DHECbottomlockcapv2 (Autodesk Fusion 360 design; units mm, degrees)
Autodesk Fusion 360 part; units mm, degrees
note: some values were not read from the file. Chosen so that the rebuilt part matches the saved one: a direction. Set by a fixed rule: which sketch regions a step uses.
sketch "Sketch1" plane through (0, 0, 0) normal (0, 0, 1) x (1, 0, 0)
  circle A0 centre (0, 0) radius 37.5
  dimension "d1" = 75
  constraint coincident A0.centre origin
  measures "d1" diameter of A0
extrude "Extrude1" add sketch "Sketch1" along normal blind 5
sketch "Sketch2" plane through (0, 0, 0) normal (1, 0, 0) x (0, 1, 0)
  line L0 (-6.5, 5) -> (-6.5, 15)
  line L1 (6.5, 5) -> (6.5, 15)
  circle A0 centre (0, 15) radius 6.5
  line L2 (0, 1.75) -> (0, 22.5)
  line L3 (37.5, 5) -> (-37.5, 5)
  line L4 (-10, 5) -> (-10, 15)
  circle A1 centre (0, 15) radius 10
  line L5 (10, 5) -> (10, 15)
  line L6 (-10, 15) -> (-6.5, 15)
  line L7 (10, 15) -> (6.5, 15)
  circle A2 centre (0, 15) radius 3.5
  dimension "d4" = 13
  dimension "d5" = 10
  dimension "d6" = 20
  dimension "d14" = 7
  constraint vertical L0
  constraint vertical L1
  constraint coincident L1.end A0
  constraint tangent L1 A0
  constraint tangent L0 A0
  constraint coincident A0.centre L2
  constraint coincident L3 L4.start
  constraint perpendicular L3 L4
  constraint concentric A0 A1
  constraint coincident L4.end A1
  constraint coincident L3 L5.start
  constraint coincident A1 L5.end
  constraint tangent A1 L5
  constraint vertical L5
  constraint horizontal L4.end A0.centre
  constraint perpendicular L0 L6
  constraint concentric A0 A2
  measures "d4" diameter of A0
  measures "d5" distance of A0.centre L3
  measures "d6" diameter of A1
  measures "d14" diameter of A2
extrude "Extrude2" add sketch "Sketch2" along normal mid plane 35 contours L0 L3 L4 A1 | L0 L3 A1 | L0 A1 L6 | L0 A0 L2 A1 | L1 L3 A1 | L1 A0 L2 A1 | L1 L3 A1 L5 | L1 A1 L7
extrude "Extrude3" add sketch "Sketch2" along normal blind 5 from surface at 17.5 contours L0 L3 L4 A1 | L0 L3 A1 | L0 A1 L6 | L0 A0 L2 A1 | L1 L3 A1 | L1 A0 L2 A1 | A0 A1 L6 L7 | A0 L2 A2 | A0 L2 A2 | L1 L3 A1 L5 | L1 A1 L7
mirror "Mirror1" about plane through (0, 0, 0) normal (1, 0, 0) of "Extrude3"
sketch "Sketch3" plane through (0, 0, 0) normal (0, 1, 0) x (1, 0, 0)
sketch "Sketch4" plane through (0, 0, 5) normal (0, 0, 1) x (-1, 0, 0)
  circle A0 centre (0, 0) radius 37.5
  line L0 (-22.5, 10) -> (22.5, 10)
  line L1 (22.5, 10) -> (22.5, -10)
  line L2 (22.5, -10) -> (-22.5, -10)
  line L3 (-22.5, -10) -> (-22.5, 10)
  circle A1 centre (0, 32.5) radius 5
  line L4 (5, 32.5) -> (5, 37.1652)
  line L5 (-5, 32.5) -> (-5, 37.1652)
  dimension "d15" = 10
  constraint tangent A0 A1
  constraint vertical A1.centre A0.centre
  constraint coincident A1 L4.start
  constraint coincident A0 L4.end
  constraint coincident A1 L5.start
  constraint coincident A0 L5.end
  constraint tangent A1 L5
  constraint tangent A1 L4
  constraint parallel L4 L5
  constraint parallel L3 L4
  measures "d15" diameter of A1
extrude "Extrude4" cut sketch "Sketch4" against normal through all contours A0 A1 L4 | A0 A1 L5 | A1
equation "d7 = ( 35 / 2 ) * 1 mm"
equation "d9 = ( 35 / 2 ) * 1 mm"
